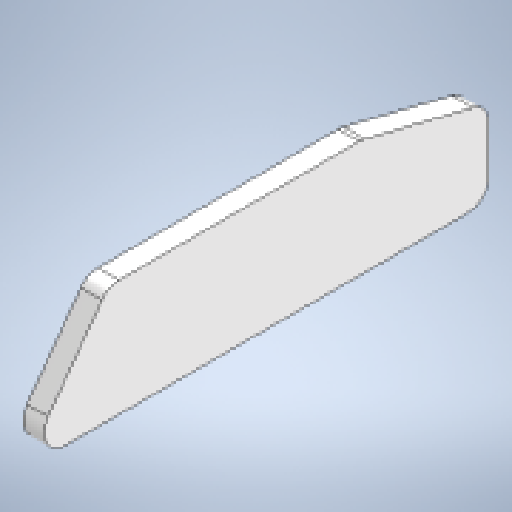
# Autodesk Inventor part: Wheel Guards
Saved by Autodesk Inventor 2023.2 (Build 272271000, 271)
## iProperties
Created: 2023-11-13
Part Number: Wheel Guards
Material: UHMW, White
Document SubType Name: Modeling
Designer: Nathan Cai
Density: 0.94 g/cm^3
Appearance: Smooth - White
Mass: 20.2324 g
Surface Area: 86.4727 cm^2
Volume: 21.5238 cm^3
Author: Nathan Cai
Autodesk Inventor part; units mm, degrees
ref_plane "YZ Plane" through (0, 0, 0) normal (1, 0, 0) x (0, 1, 0)
ref_plane "XZ Plane" through (0, 0, 0) normal (0, 1, 0) x (-1, 0, 0)
ref_plane "XY Plane" through (0, 0, 0) normal (0, 0, 1) x (1, 0, 0)
sketch "Sketch1" plane through (0, 0, 0) normal (1, 0, 0) x (0, 1, 0)
  line L0 (-17.4625, 69.85) -> (17.4625, 69.85)
  line L1 (17.4625, 69.85) -> (17.4625, -69.85)
  line L2 (17.4625, -69.85) -> (-17.4625, -69.85)
  line L3 (-17.4625, -69.85) -> (-17.4625, 69.85)
  line L4 (-17.4625, 69.85) -> (17.4625, -69.85) construction
  line L5 (17.4625, 69.85) -> (-17.4625, -69.85) construction
  line L6 (-17.4625, 69.85) -> (17.4625, 44.45)
  point P0 (0, 0)
  dimension "d0" = 34.925
  dimension "d1" = 139.7
  dimension "d2" = 25.4
  constraints: 14 end point, 2 midpoint, 2 parallel, 1 horizontal, 1 perpendicular, 1 point on line
  measures "d0" distance of L1.end L2.end
  measures "d1" distance of L0.end L1.end
  measures "d2" distance from line of L0 L6.end
extrude "Extrusion1" add sketch "Sketch1" along normal blind 6.35 contours L6 L1 L2 L3
chamfer "Chamfer1" distance 9.525 distance2 38.1 1 edges at (3.175, 17.4625, -69.85) measured on face at (3.175, 16.9625, -69.85)
fillet "Fillet1" radius 6.35 4 edges at (3.175, -17.4625, 69.85) (3.175, 17.4625, -31.75) (3.175, 7.9375, -69.85) (3.175, -17.4625, -69.85)
fillet "Fillet2" radius 6.35 1 edges at (3.175, 17.4625, 44.45)
body "Solid1"
